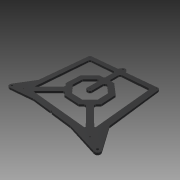
# Autodesk Inventor part: heatbed_mount_v3
Saved by Autodesk Inventor 2014 (Build 180170000, 170)
## iProperties
Created: 2013-12-04
Part Number: heatbed_mount_v3
Material: Plywood, Finish
Document SubType Name: Modeling
Designer: buben
Density: 0.552 g/cm^3
Appearance: Plywood - New
Author: buben
Subject: Laser Cutted
Autodesk Inventor part; units mm, degrees
ref_plane "YZ Plane" through (0, 0, 0) normal (1, 0, 0) x (0, 1, 0)
ref_plane "XZ Plane" through (0, 0, 0) normal (0, 1, 0) x (-1, 0, 0)
ref_plane "XY Plane" through (0, 0, 0) normal (0, 0, 1) x (1, 0, 0)
sketch "Sketch1" plane through (0, 0, 0) normal (0, 0, 1) x (1, 0, 0)
  line L0 (0, 0) -> (220, 0)
  line L1 (220, 0) -> (220, 220)
  line L2 (220, 220) -> (0, 220)
  line L3 (0, 220) -> (0, 0)
  line L4 (5.5, 214.5) -> (214.5, 214.5) construction
  line L5 (214.5, 214.5) -> (214.5, 5.5) construction
  line L6 (214.5, 5.5) -> (5.5, 5.5) construction
  line L7 (5.5, 5.5) -> (5.5, 214.5) construction
  circle A0 centre (5.5, 5.5) radius 1.6
  circle A1 centre (5.5, 214.5) radius 1.6
  circle A2 centre (214.5, 214.5) radius 1.6
  circle A3 centre (214.5, 5.5) radius 1.6
  line L8 (165, 87.2183) -> (132.7817, 55)
  line L9 (132.7817, 55) -> (87.2183, 55)
  line L10 (87.2183, 55) -> (55, 87.2183)
  line L11 (55, 87.2183) -> (55, 132.7817)
  line L12 (55, 132.7817) -> (87.2183, 165)
  line L13 (132.7817, 165) -> (165, 132.7817)
  line L14 (165, 132.7817) -> (165, 87.2183)
  line L15 (150, 126.5685) -> (150, 93.4315)
  line L16 (150, 93.4315) -> (126.5685, 70)
  line L17 (126.5685, 70) -> (93.4315, 70)
  line L18 (93.4315, 70) -> (70, 93.4315)
  line L19 (70, 93.4315) -> (70, 126.5685)
  line L20 (70, 126.5685) -> (93.4315, 150)
  line L21 (93.4315, 150) -> (126.5685, 150)
  line L22 (126.5685, 150) -> (150, 126.5685)
  line L23 (205, 205) -> (205, 15)
  line L24 (205, 15) -> (15, 15)
  line L25 (15, 15) -> (15, 205)
  line L26 (102.5, 165) -> (102.5, 205)
  line L27 (117.5, 205) -> (117.5, 165)
  line L28 (15, 205) -> (102.5, 205)
  line L29 (117.5, 205) -> (205, 205)
  line L30 (87.2183, 165) -> (102.5, 165)
  line L31 (117.5, 165) -> (132.7817, 165)
  point P0 (214.5, 110)
  point P1 (220, 110)
  point P2 (110, 214.5)
  point P3 (110, 220)
  point P4 (110, 110)
  point P5 (110, 110)
  dimension "d0" = 220
  dimension "d1" = 220
  dimension "d2" = 209
  dimension "d3" = 209
  dimension "d4" = 3.2
  dimension "d5" = 3.2
  dimension "d6" = 3.2
  dimension "d7" = 3.2
  dimension "d9" = 15
  dimension "d10" = 15
  dimension "d11" = 15
  dimension "d12" = 15
  dimension "d13" = 15
  dimension "d14" = 80
  dimension "d15" = 7.5
  constraints: 64 end point, 9 parallel, 5 coincident, 5 perpendicular, 4 centre point, 4 horizontal, 4 horizontal alignment, 4 midpoint, 2 collinear, 2 vertical alignment, 32 other
  measures "d0" distance of L0.start L0.end
  measures "d1" distance of L2.end L0.start
  measures "d2" distance of L5.end L6.end
  measures "d3" distance of L6.end L4.start
  measures "d4" diameter of A0
  measures "d5" diameter of A3
  measures "d6" diameter of A1
  measures "d7" diameter of A2
  measures "d9" distance between parallel lines of L11 L19
  measures "d10" distance between parallel lines of L3 L25
  measures "d11" distance between parallel lines of L27 L26
  measures "d12" distance between parallel lines of L1 L23
  measures "d13" distance between parallel lines of L0 L24
  measures "d14" distance between parallel lines of L15 L19
  measures "d15" distance from line of point (110, 110) L26
extrude "Extrusion1" add sketch "Sketch1" along normal blind 6.5
sketch "Sketch2" plane through (0, 0, 6.5) normal (0, 0, 1) x (1, 0, 0)
  line L0 (205, 205) -> (205, 15) projected
  line L1 (205, 15) -> (15, 15) projected
  line L2 (15, 15) -> (15, 205) projected
  line L3 (55, 87.2183) -> (87.2183, 55) projected
  line L4 (132.7817, 55) -> (165, 87.2183) projected
  line L5 (0, 220) -> (0, 0) projected
  line L6 (65.8058, 76.4124) -> (15, 25.6066)
  line L7 (76.4124, 65.8058) -> (25.6066, 15)
  line L8 (143.5876, 65.8058) -> (194.3934, 15)
  line L9 (154.1942, 76.4124) -> (205, 25.6066)
  line L10 (205, 25.6066) -> (205, 15)
  line L11 (205, 15) -> (194.3934, 15)
  line L12 (15, 25.6066) -> (15, 15)
  line L13 (15, 15) -> (25.6066, 15)
  line L14 (15, 15) -> (71.1091, 71.1091) construction
  line L15 (148.8909, 71.1091) -> (205, 15) construction
  line L16 (65.8058, 76.4124) -> (76.4124, 65.8058)
  line L17 (143.5876, 65.8058) -> (154.1942, 76.4124)
  dimension "d18" = 15
  dimension "d19" = 15
  dimension "d20" = 7.5
  dimension "d21" = 7.5
  constraints: 24 end point, 8 point on line, 4 parallel, 4 perpendicular, 3 collinear, 2 midpoint
  measures "d18" distance between parallel lines of L9 L8
  measures "d19" distance between parallel lines of L6 L7
  measures "d20" distance between parallel lines of L14 L6
  measures "d21" distance between parallel lines of L15 L8
extrude "Extrusion2" add sketch "Sketch2" against normal blind 6.5
sketch "Sketch4" plane through (0, 0, 6.5) normal (0, 0, 1) x (1, 0, 0)
  line L0 (93.4315, 150) -> (126.5685, 150) projected
  line L1 (0, 0) -> (220, 0) projected
  line L2 (220, 0) -> (220, 220) projected
  line L3 (220, 220) -> (0, 220) projected
  line L4 (0, 220) -> (0, 0) projected
  line L5 (-23.9453, -6) -> (243.9453, -6) construction
  line L6 (-23.9453, -6) -> (110, 226) construction
  line L7 (110, 226) -> (243.9453, -6) construction
  circle A0 centre (110, 226) radius 2.75
  circle A1 centre (243.9453, -6) radius 2.75
  circle A2 centre (-23.9453, -6) radius 2.75
  arc A3 (-30.4405, -2.25) -> (-22.5946, -13.3774) centre (-23.9453, -6) ccw
  arc A4 (116.4952, 229.75) -> (103.5048, 229.75) centre (110, 226) ccw
  arc A5 (242.5946, -13.3774) -> (250.4405, -2.25) centre (243.9453, -6) ccw
  line L8 (122.1244, 220) -> (116.4952, 229.75)
  line L9 (103.5048, 229.75) -> (97.8756, 220)
  line L10 (0, 50.4744) -> (-30.4405, -2.25)
  line L11 (250.4405, -2.25) -> (220, 50.4744)
  line L12 (242.5946, -13.3774) -> (169.5256, 0)
  line L13 (-22.5946, -13.3774) -> (50.4744, 0)
  line L14 (0, 50.4744) -> (0, 0)
  line L15 (0, 0) -> (50.4744, 0)
  line L16 (169.5256, 0) -> (220, 0)
  line L17 (220, 50.4744) -> (220, 0)
  point P0 (110, 150)
  dimension "d30" = 5.5
  dimension "d31" = 5.5
  dimension "d32" = 5.5
  dimension "d33" = 15
  dimension "d34" = 15
  dimension "d35" = 15
  dimension "d36" = 6
  dimension "d37" = 6
  constraints: 26 end point, 6 centre point, 6 coincident, 6 point on circle, 6 point on line, 6 tangent, 4 equal length, 4 parallel, 3 collinear, 2 perpendicular, 1 midpoint, 1 vertical alignment
  measures "d30" diameter of A1
  measures "d31" diameter of A2
  measures "d32" diameter of A0
  measures "d33" diameter of A5
  measures "d34" diameter of A3
  measures "d35" diameter of A4
  measures "d36" distance from line of L3 A0.centre
  measures "d37" distance between parallel lines of L5 L1
extrude "Extrusion3" add sketch "Sketch4" against normal blind 6.5 contours L1 L13 A3 L10 L4 | L1 L2 L11 A5 L12 | L9 A4 L8 L3
chamfer "Chamfer1" distance 4 angle 45 16 edges at (25.6066, 15, 3.25) (15, 25.6066, 3.25) (76.4124, 65.8058, 3.25) (65.8058, 76.4124, 3.25) (194.3934, 15, 3.25) (205, 25.6066, 3.25) (143.5876, 65.8058, 3.25) (154.1942, 76.4124, 3.25) (117.5, 205, 3.25) (102.5, 205, 3.25) (117.5, 165, 3.25) (102.5, 165, 3.25) (205, 205, 3.25) (15, 205, 3.25) (0, 220, 3.25) (220, 220, 3.25)
sketch "Sketch5" plane through (0, 0, 6.5) normal (0, 0, 1) x (1, 0, 0)
  line L0 (117.5, 169) -> (117.5, 201) projected
  line L1 (28.435, 17.8284) -> (29.6066, 15) projected
  line L2 (15, 29.6066) -> (17.8284, 28.435) projected
  line L3 (102.5, 201) -> (102.5, 169) projected
  line L4 (93.4315, 150) -> (126.5685, 150) projected
  line L5 (0, 216) -> (4, 220) projected
  line L6 (220, 50.4744) -> (220, 216) projected
  line L7 (70, 126.5685) -> (150, 93.4315) construction
  line L8 (150, 126.5685) -> (70, 93.4315) construction
  line L9 (102.5, 150) -> (102.5, 106)
  line L10 (102.5, 106) -> (106, 102.5)
  line L11 (106, 102.5) -> (114, 102.5)
  line L12 (114, 102.5) -> (117.5, 106)
  line L13 (117.5, 106) -> (117.5, 150)
  circle A0 centre (110, 110) radius 1.5
  point P0 (0, 0)
  dimension "d43" = 3
  dimension "d44" = 8
  dimension "d45" = 7.5
  dimension "d46" = 7.5
  constraints: 14 end point, 6 perpendicular, 2 collinear, 2 parallel, 2 point on line, 1 centre point, 1 midpoint
  measures "d43" diameter of A0
  measures "d44" distance of L10.end L11.end
  measures "d45" distance from line of L9 A0.centre
  measures "d46" distance from line of L11 A0.centre
extrude "Extrusion4" add sketch "Sketch5" against normal blind 6.5
chamfer "Chamfer2" distance 4 angle 45 2 edges at (102.5, 150, 3.25) (117.5, 150, 3.25)
sketch "Sketch6" plane through (0, 0, 6.5) normal (0, 0, 1) x (1, 0, 0)
  line L0 (50.4744, 0) -> (169.5256, 0) projected
  line L1 (107.5, 0) -> (107.5, 1.4434)
  line L2 (107.5, 1.4434) -> (110, 2.8868)
  line L3 (110, 2.8868) -> (112.5, 1.4434)
  line L4 (112.5, 1.4434) -> (112.5, 0)
  line L5 (107.5, 0) -> (112.5, 0)
  point P0 (0, 0)
  point P1 (110, 0)
  dimension "d52" = 5
  constraints: 10 end point, 2 point on line, 1 horizontal alignment, 1 midpoint, 1 perpendicular, 6 other
  measures "d52" distance between parallel lines of L4 L1
extrude "Extrusion5" cut sketch "Sketch6" against normal through all
equation "\"d5\" = d4"
equation "\"d6\" = d4"
equation "\"d7\" = d4"
equation "\"d31\" = d30"
equation "\"d32\" = d30"
equation "\"d34\" = d33"
equation "\"d35\" = d33"
equation "\"d46\" = d45"
body "Solid1"
